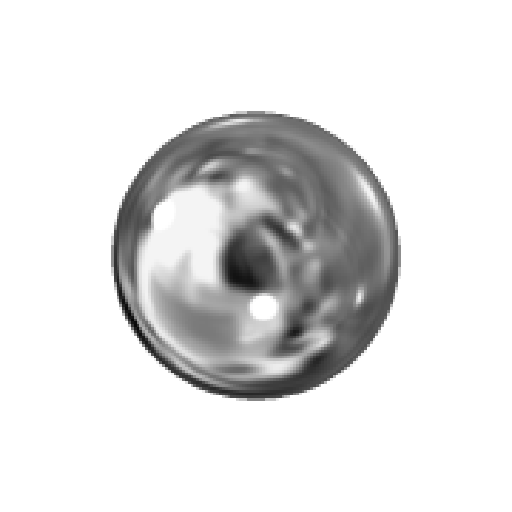
# Autodesk Inventor part: 00_Magnet_Neodym_5mm
Saved by Autodesk Inventor 2025.1 (Build 291241000, 241)
## iProperties
Created: 2024-10-22
Part Number: 00_Magnet_Neodym_5mm
Material: Generic
Document SubType Name: Modeling
Designer: Muriel
Density: 1 g/cm^3
Appearance: Chrome - Polished
Author: Muriel
Autodesk Inventor part; units mm, degrees
ref_plane "YZ Plane" through (0, 0, 0) normal (1, 0, 0) x (0, 1, 0)
ref_plane "XZ Plane" through (0, 0, 0) normal (0, 1, 0) x (-1, 0, 0)
ref_plane "XY Plane" through (0, 0, 0) normal (0, 0, 1) x (1, 0, 0)
sketch "Sketch1" plane through (0, 0, 0) normal (0, 1, 0) x (-1, 0, 0)
  circle A0 centre (0, 0) radius 2.5
  line L0 (2.5, 0) -> (-2.5, 0)
  dimension "d0" = 5
  constraints: 2 end point, 2 point on circle, 1 centre point, 1 coincident
  measures "d0" diameter of A0
revolve "Revolution1" add sketch "Sketch1" angle 360 about axis through (-2.5, 0, 0) along (1, 0, 0) picked at (0.6238, 0.5526) contours L0 A0
body "Solid1"
